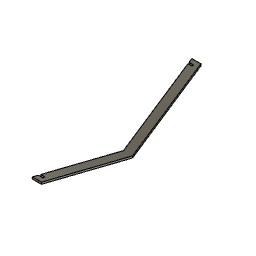
Lampi1 (Autodesk Fusion 360 design; units mm, degrees)
Autodesk Fusion 360 part; units mm, degrees
note: some values were not read from the file. Set by a fixed rule: which sketch regions a step uses.
sketch "Sketch1" plane through (0, 0, 0) normal (0, 0, 1) x (1, 0, 0)
  line L0 (0, 0) -> (20, 0)
  line L1 (20, 0) -> (120, -250)
  line L2 (120, -250) -> (70, -400)
  line L3 (70, -400) -> (50, -400)
  line L4 (4, -10) -> (14, -10)
  line L5 (53.3333, -390) -> (63.3333, -390)
  line L6 (63.3333, -386) -> (54.6667, -386)
  line L7 (100, -250) -> (54.6667, -386)
  line L8 (53.3333, -390) -> (50, -400)
  line L9 (0, 0) -> (4, -10)
  line L10 (5.6, -14) -> (100, -250)
  line L11 (14, -10) -> (14, -14)
  line L12 (5.6, -14) -> (14, -14)
  line L13 (63.3333, -390) -> (63.3333, -386)
  dimension "d4" = 400
  dimension "d5" = 50
  dimension "d6" = 50
  dimension "d7" = 250
  dimension "d9" = 20
  dimension "d10" = 20
  dimension "d11" = 20
  dimension "d12" = 10
  dimension "d13" = 4
  dimension "d14" = 10
  dimension "d15" = 10
  dimension "d16" = 4
  dimension "d17" = 10
  dimension "d27" = 4
  constraint coincident L0.start L9.start
  constraint horizontal L0
  constraint parallel L0 L3
  constraint parallel L1 L9
  constraint parallel L0 L4
  constraint coincident L10.start L9
  constraint coincident L5.start L7
  constraint parallel L3 L5
  constraint parallel L5 L6
  constraint collinear L7 L8
  constraint collinear L9 L10
  constraint perpendicular L11 L12
  constraint perpendicular L6 L13
  measures "d4" vertical distance of L0.start L3.end
  measures "d5" horizontal distance of L7.start L3.end
  measures "d6" horizontal distance of L0.start L3.end
  measures "d7" vertical distance of L0.start L7.start
  measures "d9" distance of L0.start L0.end
  measures "d10" distance of L7.start L1.end
  measures "d11" horizontal distance of L3.end L2.end
  measures "d12" vertical distance of L0.start L4.start
  measures "d13" vertical distance of L4.start L10.start
  measures "d14" distance of L4.start L4.end
  measures "d15" vertical distance of L3.end L5.start
  measures "d16" vertical distance of L5.start L6.end
  measures "d17" distance of L5.start L5.end
  measures "d27" distance of L4.end L11.end
extrude "Extrude1" add sketch "Sketch1" along normal blind 4
sketch "Sketch1 (2)" plane through (0, 0, 0) normal (0, 0, 1) x (1, 0, 0) in component "Lampi1"
component "Lampi1" placed x (1, 0, 0) y (0, 1, 0) z (0, 0, 1) at (0, 0, 0)
equation "d4 = haed_skerms"
equation "d5 = umfram_radius"
equation "d6 = umfram_radius"
equation "d7 = haed_u"
equation "d9 = þykkt_eining"
equation "d10 = þykkt_eining"
equation "d11 = þykkt_eining"
equation "d12 = dypt_pressfit"
equation "d13 = þykkt"
equation "d14 = dypt_pressfit"
equation "d15 = dypt_pressfit"
equation "d16 = þykkt"
equation "d17 = dypt_pressfit"
equation "haed_skerms = 400 mm"
equation "haed_u = 250 mm"
equation "head_l = 150 mm"
equation "þykkt = 4 mm"
equation "dypt_pressfit = 10 mm"
equation "umfram_radius = 50 mm"
equation "þykkt_eining = 20 mm"
